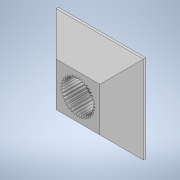
# Autodesk Inventor part: Servo Grip
Saved by Autodesk Inventor 2020.2 (Build 242310000, 310)
## iProperties
Created: 2020-03-15
Part Number: Servo Grip
Material: Generic
Document SubType Name: Modeling
Designer: Varun Kumar
Density: 1 g/cm^3
Appearance: Default
Author: Varun Kumar
Autodesk Inventor part; units mm, degrees
ref_plane "YZ Plane" through (0, 0, 0) normal (1, 0, 0) x (0, 1, 0)
ref_plane "XZ Plane" through (0, 0, 0) normal (0, 1, 0) x (-1, 0, 0)
ref_plane "XY Plane" through (0, 0, 0) normal (0, 0, 1) x (1, 0, 0)
sketch "Sketch1" plane through (0, 0, 0) normal (0, 0, 1) x (1, 0, 0)
  line L0 (-6.35, -6.35) -> (6.35, -6.35)
  line L1 (6.35, -6.35) -> (6.35, 6.35)
  line L2 (6.35, 6.35) -> (-6.35, 6.35)
  line L3 (-6.35, 6.35) -> (-6.35, -6.35)
  line L4 (-6.35, -6.35) -> (6.35, 6.35) construction
  line L5 (6.35, -6.35) -> (-6.35, 6.35) construction
  line L6 (-0.3534, 2.4749) -> (-0.4996, 2.1425)
  line L7 (-0.3534, 2.4749) -> (-0.12, 2.1967)
  line L8 (-0.7778, 2.3759) -> (-0.8641, 2.0232)
  line L9 (-0.7778, 2.3759) -> (-0.4996, 2.1425)
  line L10 (-1.1786, 2.2048) -> (-1.2023, 1.8424)
  line L11 (-1.1786, 2.2048) -> (-0.8641, 2.0232)
  line L12 (-1.5435, 1.9666) -> (-1.504, 1.6056)
  line L13 (-1.5435, 1.9666) -> (-1.2023, 1.8424)
  line L14 (-1.8616, 1.6687) -> (-1.7599, 1.3201)
  line L15 (-1.8616, 1.6687) -> (-1.504, 1.6056)
  line L16 (-2.1231, 1.3201) -> (-1.9624, 0.9944)
  line L17 (-2.1231, 1.3201) -> (-1.7599, 1.3201)
  line L18 (-2.32, 0.9314) -> (-2.1053, 0.6386)
  line L19 (-2.32, 0.9314) -> (-1.9624, 0.9944)
  line L20 (-2.4465, 0.5144) -> (-2.1842, 0.2633)
  line L21 (-2.4465, 0.5144) -> (-2.1053, 0.6386)
  line L22 (-2.4987, 0.0817) -> (-2.1967, -0.12)
  line L23 (-2.4987, 0.0817) -> (-2.1842, 0.2633)
  line L24 (-2.4749, -0.3534) -> (-2.1425, -0.4996)
  line L25 (-2.4749, -0.3534) -> (-2.1967, -0.12)
  line L26 (-2.3759, -0.7778) -> (-2.0232, -0.8641)
  line L27 (-2.3759, -0.7778) -> (-2.1425, -0.4996)
  line L28 (-2.2048, -1.1786) -> (-1.8424, -1.2023)
  line L29 (-2.2048, -1.1786) -> (-2.0232, -0.8641)
  line L30 (-1.9666, -1.5435) -> (-1.6056, -1.504)
  line L31 (-1.9666, -1.5435) -> (-1.8424, -1.2023)
  line L32 (-1.6687, -1.8616) -> (-1.3201, -1.7599)
  line L33 (-1.6687, -1.8616) -> (-1.6056, -1.504)
  line L34 (-1.3201, -2.1231) -> (-0.9944, -1.9624)
  line L35 (-1.3201, -2.1231) -> (-1.3201, -1.7599)
  line L36 (-0.9314, -2.32) -> (-0.6386, -2.1053)
  line L37 (-0.9314, -2.32) -> (-0.9944, -1.9624)
  line L38 (-0.5144, -2.4465) -> (-0.2633, -2.1842)
  line L39 (-0.5144, -2.4465) -> (-0.6386, -2.1053)
  line L40 (-0.0817, -2.4987) -> (0.12, -2.1967)
  line L41 (-0.0817, -2.4987) -> (-0.2633, -2.1842)
  line L42 (0.3534, -2.4749) -> (0.4996, -2.1425)
  line L43 (0.3534, -2.4749) -> (0.12, -2.1967)
  line L44 (0.7778, -2.3759) -> (0.8641, -2.0232)
  line L45 (0.7778, -2.3759) -> (0.4996, -2.1425)
  line L46 (1.1786, -2.2048) -> (1.2023, -1.8424)
  line L47 (1.1786, -2.2048) -> (0.8641, -2.0232)
  line L48 (1.5435, -1.9666) -> (1.504, -1.6056)
  line L49 (1.5435, -1.9666) -> (1.2023, -1.8424)
  line L50 (1.8616, -1.6687) -> (1.7599, -1.3201)
  line L51 (1.8616, -1.6687) -> (1.504, -1.6056)
  line L52 (2.1231, -1.3201) -> (1.9624, -0.9944)
  line L53 (2.1231, -1.3201) -> (1.7599, -1.3201)
  line L54 (2.32, -0.9314) -> (2.1053, -0.6386)
  line L55 (2.32, -0.9314) -> (1.9624, -0.9944)
  line L56 (2.4465, -0.5144) -> (2.1842, -0.2633)
  line L57 (2.4465, -0.5144) -> (2.1053, -0.6386)
  line L58 (2.4987, -0.0817) -> (2.1967, 0.12)
  line L59 (2.4987, -0.0817) -> (2.1842, -0.2633)
  line L60 (2.4749, 0.3534) -> (2.1425, 0.4996)
  line L61 (2.4749, 0.3534) -> (2.1967, 0.12)
  line L62 (2.3759, 0.7778) -> (2.0232, 0.8641)
  line L63 (2.3759, 0.7778) -> (2.1425, 0.4996)
  line L64 (2.2048, 1.1786) -> (1.8424, 1.2023)
  line L65 (2.2048, 1.1786) -> (2.0232, 0.8641)
  line L66 (1.9666, 1.5435) -> (1.6056, 1.504)
  line L67 (1.9666, 1.5435) -> (1.8424, 1.2023)
  line L68 (1.6687, 1.8616) -> (1.3201, 1.7599)
  line L69 (1.6687, 1.8616) -> (1.6056, 1.504)
  line L70 (1.3201, 2.1231) -> (0.9944, 1.9624)
  line L71 (1.3201, 2.1231) -> (1.3201, 1.7599)
  line L72 (0.9314, 2.32) -> (0.6386, 2.1053)
  line L73 (0.9314, 2.32) -> (0.9944, 1.9624)
  line L74 (0.5144, 2.4465) -> (0.2633, 2.1842)
  line L75 (0.5144, 2.4465) -> (0.6386, 2.1053)
  line L76 (0.0817, 2.4987) -> (-0.12, 2.1967)
  line L77 (0.0817, 2.4987) -> (0.2633, 2.1842)
  circle A0 centre (0, 0) radius 0.3723
  point P0 (0, 0)
  dimension "d0" = 12.7
  dimension "d1" = 12.7
  constraints: 156 end point, 2 midpoint, 2 parallel, 1 centre point, 1 horizontal, 1 perpendicular
  measures "d0" distance of L2.end L1.end
  measures "d1" distance of L1.end L0.end
extrude "Extrusion1" add sketch "Sketch1" along normal blind 3.5 contours L3 L2 L1 L0 | L7 L76 L77 L74 L75 L72 L73 L70 L71 L68 L69 L66 L67 L64 L65 L62 L63 L60 L61 L58 L59 L56 L57 L54 L55 L52 L53 L50 L51 L48 L49 L46 L47 L44 L45 L42 L43 L40 L41 L38 L39 L36 L37 L34 L35 L32 L33 L30 L31 L28 L29 L26 L27 L24 L25 L22 L23 L20 L21 L18 L19 L16 L17 L14 L15 L12 L13 L10 L11 L8 L9 L6 | A0
sketch "Sketch2" plane through (0, 0, 3.5) normal (0, 0, 1) x (1, 0, 0)
  line L0 (2.2048, 1.1786) -> (1.8424, 1.2023)
  line L1 (2.2048, 1.1786) -> (2.0232, 0.8641)
  line L2 (2.4749, 0.3534) -> (2.1425, 0.4996)
  line L3 (2.4749, 0.3534) -> (2.1967, 0.12)
  line L4 (2.4987, -0.0817) -> (2.1967, 0.12)
  line L5 (2.4987, -0.0817) -> (2.1842, -0.2633)
  line L6 (-0.3534, 2.4749) -> (-0.12, 2.1967)
  line L7 (-0.3534, 2.4749) -> (-0.4996, 2.1425)
  line L8 (-1.5435, 1.9666) -> (-1.504, 1.6056)
  line L9 (-1.8616, 1.6687) -> (-1.504, 1.6056)
  line L10 (-1.8616, 1.6687) -> (-1.7599, 1.3201)
  line L11 (-1.5435, 1.9666) -> (-1.2023, 1.8424)
  line L12 (-1.1786, 2.2048) -> (-1.2023, 1.8424)
  line L13 (-1.1786, 2.2048) -> (-0.8641, 2.0232)
  line L14 (-0.7778, 2.3759) -> (-0.8641, 2.0232)
  line L15 (-0.7778, 2.3759) -> (-0.4996, 2.1425)
  line L16 (-2.1231, 1.3201) -> (-1.7599, 1.3201)
  line L17 (-2.1231, 1.3201) -> (-1.9624, 0.9944)
  line L18 (-2.32, 0.9314) -> (-1.9624, 0.9944)
  line L19 (-2.32, 0.9314) -> (-2.1053, 0.6386)
  line L20 (-2.4465, 0.5144) -> (-2.1053, 0.6386)
  line L21 (-2.4465, 0.5144) -> (-2.1842, 0.2633)
  line L22 (-2.4987, 0.0817) -> (-2.1842, 0.2633)
  line L23 (-2.4987, 0.0817) -> (-2.1967, -0.12)
  line L24 (-2.4749, -0.3534) -> (-2.1967, -0.12)
  line L25 (-2.4749, -0.3534) -> (-2.1425, -0.4996)
  line L26 (-2.3759, -0.7778) -> (-2.1425, -0.4996)
  line L27 (-2.3759, -0.7778) -> (-2.0232, -0.8641)
  line L28 (-2.2048, -1.1786) -> (-2.0232, -0.8641)
  line L29 (-2.2048, -1.1786) -> (-1.8424, -1.2023)
  line L30 (-1.9666, -1.5435) -> (-1.8424, -1.2023)
  line L31 (-1.9666, -1.5435) -> (-1.6056, -1.504)
  line L32 (-1.6687, -1.8616) -> (-1.6056, -1.504)
  line L33 (-1.6687, -1.8616) -> (-1.3201, -1.7599)
  line L34 (-1.3201, -2.1231) -> (-1.3201, -1.7599)
  line L35 (-1.3201, -2.1231) -> (-0.9944, -1.9624)
  line L36 (-0.9314, -2.32) -> (-0.9944, -1.9624)
  line L37 (-0.9314, -2.32) -> (-0.6386, -2.1053)
  line L38 (-0.5144, -2.4465) -> (-0.6386, -2.1053)
  line L39 (-0.5144, -2.4465) -> (-0.2633, -2.1842)
  line L40 (-0.0817, -2.4987) -> (-0.2633, -2.1842)
  line L41 (-0.0817, -2.4987) -> (0.12, -2.1967)
  line L42 (0.3534, -2.4749) -> (0.12, -2.1967)
  line L43 (0.3534, -2.4749) -> (0.4996, -2.1425)
  line L44 (0.7778, -2.3759) -> (0.4996, -2.1425)
  line L45 (0.7778, -2.3759) -> (0.8641, -2.0232)
  line L46 (1.1786, -2.2048) -> (0.8641, -2.0232)
  line L47 (1.1786, -2.2048) -> (1.2023, -1.8424)
  line L48 (1.5435, -1.9666) -> (1.2023, -1.8424)
  line L49 (1.5435, -1.9666) -> (1.504, -1.6056)
  line L50 (1.8616, -1.6687) -> (1.504, -1.6056)
  line L51 (1.8616, -1.6687) -> (1.7599, -1.3201)
  line L52 (2.1231, -1.3201) -> (1.7599, -1.3201)
  line L53 (2.1231, -1.3201) -> (1.9624, -0.9944)
  line L54 (2.32, -0.9314) -> (1.9624, -0.9944)
  line L55 (2.32, -0.9314) -> (2.1053, -0.6386)
  line L56 (2.4465, -0.5144) -> (2.1053, -0.6386)
  line L57 (2.4465, -0.5144) -> (2.1842, -0.2633)
  line L58 (2.3759, 0.7778) -> (2.0232, 0.8641)
  line L59 (2.3759, 0.7778) -> (2.1425, 0.4996)
  line L60 (1.9666, 1.5435) -> (1.8424, 1.2023)
  line L61 (1.9666, 1.5435) -> (1.6056, 1.504)
  line L62 (1.6687, 1.8616) -> (1.6056, 1.504)
  line L63 (1.6687, 1.8616) -> (1.3201, 1.7599)
  line L64 (0.0817, 2.4987) -> (-0.12, 2.1967)
  line L65 (0.0817, 2.4987) -> (0.2633, 2.1842)
  circle A0 centre (0, 0) radius 0.3723
  line L66 (0.5144, 2.4465) -> (0.2633, 2.1842)
  line L67 (0.5144, 2.4465) -> (0.6386, 2.1053)
  line L68 (1.3201, 2.1231) -> (1.3201, 1.7599)
  line L69 (1.3201, 2.1231) -> (0.9944, 1.9624)
  line L70 (0.9314, 2.32) -> (0.9944, 1.9624)
  line L71 (0.9314, 2.32) -> (0.6386, 2.1053)
  point P0 (0, 0)
  constraints: 144 end point, 1 centre point
extrude "Extrusion2" cut sketch "Sketch2" against normal blind 3.2 contours L1 L58 L59 L2 L3 L4 L5 L57 L56 L55 L54 L53 L52 L51 L50 L49 L48 L47 L46 L45 L44 L43 L42 L41 L40 L39 L38 L37 L36 L35 L34 L33 L32 L31 L30 L29 L28 L27 L26 L25 L24 L23 L22 L21 L20 L19 L18 L17 L16 L10 L9 L8 L11 L12 L13 L14 L15 L7 L6 L64 L65 L66 L67 L71 L70 L69 L68 L63 L62 L61 L60 L0 | A0
chamfer "Chamfer1" distance 3.175 angle 45 4 edges at (0, -6.35, 3.5) (-6.35, 0, 3.5) (6.35, 0, 3.5) (0, 6.35, 3.5)
body "Solid1"
